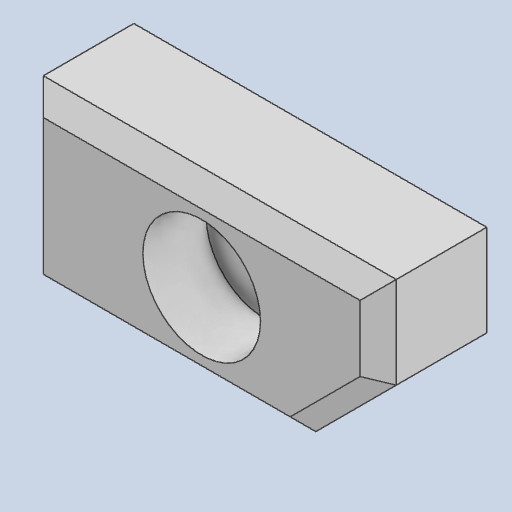
# Autodesk Inventor part: leg2
Saved by Autodesk Inventor 2022 (Build 260153000, 153)
## iProperties
Created: 2024-07-10
Part Number: leg2
Material: Типовые
Document SubType Name: Modeling
Designer: Капустяник Андрей
Density: 1 g/cm^3
Appearance: По умолчанию
Author: Капустяник Андрей
Autodesk Inventor part; units mm, degrees
ref_plane "YZ Plane" through (0, 0, 0) normal (1, 0, 0) x (0, 1, 0)
ref_plane "XZ Plane" through (0, 0, 0) normal (0, 1, 0) x (-1, 0, 0)
ref_plane "XY Plane" through (0, 0, 0) normal (0, 0, 1) x (1, 0, 0)
sketch "Эскиз1" plane through (0, 0, 0) normal (0, 0, 1) x (1, 0, 0)
  line L0 (10, 5) -> (10, -0.4101) projected
  line L1 (-10, 5) -> (10, 5) projected
  line L2 (-10, -5) -> (-10, 5) projected
  line L3 (5.4101, -5) -> (-10, -5) projected
  line L4 (10, -0.4101) -> (5.4101, -5) projected
  line L5 (9.75, -0.3065) -> (9.75, 4.75)
  line L6 (9.75, 4.75) -> (-9.75, 4.75)
  line L7 (-9.75, 4.75) -> (-9.75, -4.75)
  line L8 (-9.75, -4.75) -> (5.3065, -4.75)
  line L9 (5.3065, -4.75) -> (9.75, -0.3065)
  circle A0 centre (0, 0) radius 1.6 projected
  line L10 (10, 5) -> (10, -0.4101) projected
  line L11 (-10, 5) -> (10, 5) projected
  line L12 (-10, -5) -> (-10, 5) projected
  line L13 (5.4101, -5) -> (-10, -5) projected
  line L14 (10, -0.4101) -> (5.4101, -5) projected
  circle A1 centre (0, 0) radius 1.6 projected
  dimension "d0" = 0.25
  constraints: 10 end point, 4 other
  measures "d0" distance between parallel lines of L0 L5
extrude "Выдавливание1" add sketch "Эскиз1" along normal blind 6 contours L9 L8 L7 L6 L5
chamfer "Фаска1" distance 1 angle 45 5 edges at (-2.2218, -4.75, 6) (7.5282, -2.5282, 6) (9.75, 2.2218, 6) (0, 4.75, 6) (-9.75, 0, 6)
sketch "Эскиз2" plane through (0, 0, 6) normal (0, 0, 1) x (1, 0, 0)
  circle A0 centre (0, 0) radius 3.25
  dimension "d6" = 6.5
  constraints: 1 centre point, 1 coincident
  measures "d6" diameter of A0
extrude "Выдавливание2" cut sketch "Эскиз2" against normal blind 3.5
